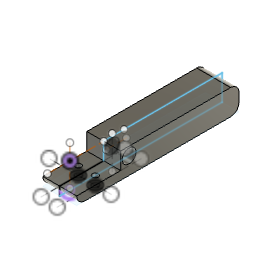
bending_tool_lever v2 (Autodesk Fusion 360 design; units mm, degrees)
Autodesk Fusion 360 part; units mm, degrees
note: some values were not read from the file. Set by a fixed rule: which sketch regions a step uses.
sketch "Skizze4" plane through (0, 0, 0) normal (0, 0, 1) x (1, 0, 0)
  line L0 (1.5, -6) -> (-1.5, -6)
  line L1 (-1.5, -6) -> (-1.5, 0)
  line L2 (-1.5, 0) -> (1.5, 0)
  line L3 (1.5, 0) -> (1.5, -6)
  line L4 (1.5, -6) -> (-1.5, 0) construction
  line L5 (-1.5, -6) -> (1.5, 0) construction
  line L6 (0, 9.7025) -> (0, -8.7035) construction
  line L7 (-7.2352, -6) -> (6.1757, -6) construction
  point P0 (0, -3)
  point P1 (0, -6)
  dimension "d21" = 3
  dimension "d22" = 6
  constraint horizontal L0
  constraint perpendicular L0 L1
  constraint parallel L0 L2
  constraint parallel L1 L3
  constraint coincident L4 P0
  constraint coincident L5 P0
  constraint vertical L6
  constraint coincident origin L6
  constraint coincident P0 L6
  constraint coincident origin L2
  constraint horizontal L7
  constraint coincident L6 P1
  constraint coincident L7 P1
  constraint coincident L0 P1
  measures "d21" distance of L0.start L0.end
  measures "d22" distance of origin L7
ref_plane "Arbeitsebene1" through (0, 0, -6.5) normal (0, 0, 1) x (1, 0, 0)
sketch "Skizze7" plane through (0, 0, -6.5) normal (0, 0, 1) x (1, 0, 0)
  line L0 (-16.0259, 10) -> (20, 10) construction
  line L1 (-5, 21.68) -> (-5, -11.619) construction
  line L2 (5, 22.2413) -> (5, -12.5543) construction
  line L3 (-2.05, 11.7032) -> (-5, 13.4064)
  line L4 (-5, 13.4064) -> (-7.95, 11.7032)
  line L5 (-7.95, 11.7032) -> (-7.95, 8.2968)
  line L6 (-7.95, 8.2968) -> (-5, 6.5936)
  line L7 (-5, 6.5936) -> (-2.05, 8.2968)
  line L8 (-2.05, 8.2968) -> (-2.05, 11.7032)
  line L9 (7.95, 11.7032) -> (5, 13.4064)
  line L10 (5, 13.4064) -> (2.05, 11.7032)
  line L11 (2.05, 11.7032) -> (2.05, 8.2968)
  line L12 (2.05, 8.2968) -> (5, 6.5936)
  line L13 (5, 6.5936) -> (7.95, 8.2968)
  line L14 (7.95, 8.2968) -> (7.95, 11.7032)
  line L15 (-15.7752, 15) -> (18.7006, 15) construction
  line L16 (0, 22.633) -> (0, -9.7229) construction
  line L17 (2.95, 16.7032) -> (0, 18.4064)
  line L18 (0, 18.4064) -> (-2.95, 16.7032)
  line L19 (-2.95, 16.7032) -> (-2.95, 13.2968)
  line L20 (-2.95, 13.2968) -> (0, 11.5936)
  line L21 (0, 11.5936) -> (2.95, 13.2968)
  line L22 (2.95, 13.2968) -> (2.95, 16.7032)
  point P0 (-5, 10)
  point P1 (5, 10)
  point P2 (-5, 10)
  point P3 (5, 10)
  point P4 (0, 15)
  point P5 (0, 15)
  dimension "d47" = 5.9
  dimension "d48" = 5.9
  dimension "d51" = 15
  dimension "d52" = 5.9
  dimension "d117" = 10
  dimension "d118" = 5
  dimension "d119" = 5
  constraint horizontal L0
  constraint vertical L1
  constraint vertical L2
  constraint coincident L0 P2
  constraint coincident L1 P2
  constraint coincident L2 P3
  constraint coincident L0 P3
  constraint coincident P2 P0
  constraint coincident P3 P1
  constraint horizontal L15
  constraint vertical L16
  constraint coincident origin L16
  constraint coincident L15 P5
  constraint coincident L16 P5
  constraint coincident P5 P4
  measures "d47" distance of L11 L14
  measures "d48" distance of L5 L8
  measures "d51" distance of origin L15
  measures "d52" distance of L19 L22
  measures "d117" distance of origin L0
  measures "d118" distance of origin L2
  measures "d119" distance of origin L1
sketch "Skizze1" plane through (0, 0, 0) normal (1, 0, 0) x (0, 1, 0) in component "Unterteil"
  line L0 (0, 9.24) -> (0, -14) construction
  line L1 (-13.3055, 0) -> (32, 0) construction
  line L2 (-6, -10) -> (20, -10)
  line L3 (20, -10) -> (20, 0)
  line L4 (90, 0) -> (90, -15)
  line L5 (90, -15) -> (-6, -15)
  line L6 (-6, -15) -> (-6, -10)
  line L7 (90, 0) -> (20, 0)
  line L8 (25, 1.4735) -> (25, -18) construction
  line L9 (33.3576, -5) -> (21.4671, -5) construction
  circle A0 centre (25, -5) radius 4.1
  dimension "d60" = 70
  dimension "d61" = 15
  dimension "d64" = 8.2
  dimension "d120" = 25
  dimension "d121" = 5
  dimension "d122" = 15
  dimension "d123" = 10
  dimension "d124" = 20
  dimension "d125" = 6
  constraint vertical L0
  constraint horizontal L1
  constraint horizontal L2
  constraint coincident L1 L3.end
  constraint perpendicular L1 L4
  constraint perpendicular L4 L5
  constraint perpendicular L5 L6
  constraint coincident L2.start L6
  constraint coincident L2.start L6.end
  constraint perpendicular L5 L8
  constraint perpendicular L3 L9
  constraint coincident L9 A0.centre
  constraint coincident L8 A0.centre
  measures "d60" distance of L4 L3.end
  measures "d61" distance of L4.start L5
  measures "d64" diameter of A0
  measures "d120" distance of origin L8
  measures "d121" vertical distance of origin A0.centre
  measures "d122" distance of L5 L7
  measures "d123" distance of origin L2
  measures "d124" distance of origin L3
  measures "d125" distance of origin L6
extrude "Extrusion1" add sketch "Skizze1" along normal mid plane 20 in component "Unterteil"
sketch "Skizze2" plane through (0, 0, -15) normal (0, 0, -1) x (1, 0, 0) in component "Unterteil"
  line L0 (-10, -90) -> (10, -90)
  line L1 (10, -90) -> (10, 6)
  line L2 (10, 6) -> (-10, 6)
  line L3 (-10, 6) -> (-10, -90)
  line L4 (14.3477, -10) -> (-22.3478, -10) construction
  line L5 (5, -37) -> (5, 12.4856) construction
  line L6 (-5, -37.5119) -> (-5, 12) construction
  circle A0 centre (-5, -10) radius 1.75
  circle A1 centre (5, -10) radius 1.75
  circle A2 centre (5, -10) radius 3.5
  circle A3 centre (-5, -10) radius 3.5
  dimension "d67" = 16
  dimension "d68" = 5
  dimension "d69" = 5
  dimension "d70" = 3.5
  dimension "d71" = 3.5
  dimension "d72" = 7
  dimension "d73" = 7
  constraint horizontal L4
  constraint vertical L5
  constraint vertical L6
  constraint coincident L4 A0.centre
  constraint coincident L6 A0.centre
  constraint coincident L4 A1.centre
  constraint coincident L5 A1.centre
  constraint concentric A1 A2
  constraint concentric A0 A3
  measures "d67" distance of L2.end L4
  measures "d68" distance of L5 origin
  measures "d69" distance of origin L6
  measures "d70" diameter of A0
  measures "d71" diameter of A1
  measures "d72" diameter of A2
  measures "d73" diameter of A3
extrude "Extrusion2" cut sketch "Skizze2" against normal blind 10 contours A0 | A1 in component "Unterteil"
extrude "Extrusion3" cut sketch "Skizze2" against normal blind 2 contours A2 | A3 in component "Unterteil"
fillet "Abrundung3" radius 5 1 edges at (0, -6, -15) in component "Unterteil"
fillet "Abrundung4" radius 5 1 edges at (0, 90, 0) in component "Unterteil"
fillet "Abrundung5" radius 5 1 edges at (0, 90, -15) in component "Unterteil"
component "Unterteil" placed x (1, 0, 0) y (0, 1, 0) z (0, 0, 1) at (0, 0, 0)
component "Basis" placed x (1, 0, 0) y (0, 1, 0) z (0, 0, 1) at (0, 0, 0)
